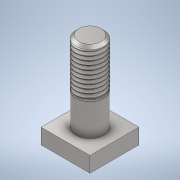
# Autodesk Inventor part: Perno de Sujeción
Saved by Autodesk Inventor 2020 (Build 240168000, 168)
## iProperties
Created: 2020-09-17
Part Number: Perno de Sujeción
Material: Steel AISI 1020 107 HR
Document SubType Name: Modeling
Designer: aaron
Density: 7.87 g/cm^3
Appearance: Stainless - Brushed
Author: aaron
Autodesk Inventor part; units mm, degrees
ref_plane "YZ Plane" through (0, 0, 0) normal (1, 0, 0) x (0, 1, 0)
ref_plane "XZ Plane" through (0, 0, 0) normal (0, 1, 0) x (-1, 0, 0)
ref_plane "XY Plane" through (0, 0, 0) normal (0, 0, 1) x (1, 0, 0)
sketch "Sketch1" plane through (0, 0, 0) normal (0, 1, 0) x (-1, 0, 0)
  line L0 (13.8906, 13.8906) -> (-13.8906, 13.8906)
  line L1 (-13.8906, 13.8906) -> (-13.8906, -13.8906)
  line L2 (-13.8906, -13.8906) -> (13.8906, -13.8906)
  line L3 (13.8906, -13.8906) -> (13.8906, 13.8906)
  line L4 (13.8906, 13.8906) -> (-13.8906, -13.8906) construction
  line L5 (-13.8906, 13.8906) -> (13.8906, -13.8906) construction
  point P0 (0, 0)
  dimension "d0" = 27.7812
  constraints: 12 end point, 2 midpoint, 2 parallel, 2 perpendicular, 1 horizontal
  measures "d0" distance of L1.end L2.end
extrude "Extrusion1" add sketch "Sketch1" against normal blind 8.7313
sketch "Sketch2" plane through (0, 0, 0) normal (0, 1, 0) x (1, 0, 0)
  circle A0 centre (0, 0) radius 7.9375
  dimension "d4" = 15.875
  constraints: 1 centre point, 1 coincident
  measures "d4" diameter of A0
extrude "Extrusion2" add sketch "Sketch2" along normal blind 45.2437
chamfer "Chamfer1" distance 1.5875 angle 45 1 edges at (-7.9375, 45.2437, 0) measured on face at (7.8347, 30.1625, 1.2733)
thread "Thread1" size "5/8-11 UNC" class "2A" standard "ANSI Unified Screw Threads" length 25.4
sketch "Sketch4" plane through (0, 43.6562, 0) normal (1, 0, 0) x (0, 0, 1)
  line L0 (7.9375, 0) -> (7.9375, 25.4)
  line L1 (7.9375, 25.4) -> (6.2254, 25.4)
  line L2 (6.2254, 25.4) -> (6.2254, 0)
  line L3 (6.2254, 0) -> (7.9375, 0)
  line L4 (0, -13.499) -> (0, 63.3686) projected
  constraints: 8 end point
revolve "Revolution1" cut sketch "Sketch4" angle 360 about axis through (0, 43.6562, 0) along (0, -1, 0)
sketch "Sketch5" plane through (0, 43.6562, 0) normal (1, 0, 0) x (0, 0, 1)
  line L0 (7.9375, 0) -> (7.9375, 25.4)
  line L1 (7.9375, 25.4) -> (6.2254, 25.4)
  line L2 (6.2254, 25.4) -> (6.2254, 0)
  line L3 (6.2254, 0) -> (7.9375, 0)
  line L4 (0, -13.499) -> (0, 63.3686) projected
  constraints: 8 end point
revolve "Revolution2" add sketch "Sketch5" angle 360 about axis through (0, 43.6562, 0) along (0, -1, 0) separate body
sketch "Sketch3" plane through (0, 43.6562, 0) normal (-1, 0, 0) x (0, -1, 0)
  line L0 (-1.3471, -6.3423) -> (-1.1546, -6.3423) construction
  line L1 (0.1923, -7.8209) -> (-0.0001, -8.1905) construction
  line L2 (-2.3092, -8.1905) -> (-2.5016, -7.8209) construction
  line L3 (-0.9622, -6.3423) -> (-1.1546, -5.9727) construction
  line L4 (-1.1546, -5.9727) -> (-1.3471, -6.3423) construction
  line L5 (-2.3092, -8.1905) -> (-2.1168, -7.8209) construction
  line L6 (-0.9622, -6.3423) -> (-0.1925, -7.8209)
  line L7 (-2.5016, -7.8209) -> (-2.1168, -7.8209) construction
  arc A0 (-2.5016, -7.8209) -> (-2.3092, -7.9377) centre (-2.3092, -7.7207) ccw construction
  line L8 (0.1923, -7.8209) -> (-0.1925, -7.8209) construction
  line L9 (-2.3092, -8.1905) -> (-2.3092, -7.8209) construction
  line L10 (-0.0001, -8.1905) -> (-0.0001, -7.8209) construction
  line L11 (-1.1546, -5.9727) -> (-1.1546, -6.2256) construction
  line L12 (-2.3092, -7.9377) -> (-0.0001, -7.9377)
  arc A1 (-2.3092, -7.9377) -> (-2.1168, -7.8209) centre (-2.3092, -7.7207) ccw
  line L13 (-0.1925, -7.8209) -> (-0.0001, -8.1905) construction
  line L14 (-2.1168, -7.8209) -> (-1.3471, -6.3423)
  line L15 (-0.0001, -0.0002) -> (-0.0001, 0.0177)
  line L16 (-0.0001, 0.0177) -> (-0.0001, -0.0002)
  line L17 (-0.0001, -0.0002) -> (0.0334, -0.0002)
  arc A2 (-0.1925, -7.8209) -> (-0.0001, -7.9377) centre (-0.0001, -7.7207) ccw
  arc A3 (-0.0001, -7.9377) -> (0.1923, -7.8209) centre (-0.0001, -7.7207) ccw construction
  arc A4 (-1.1546, -6.2256) -> (-1.3471, -6.3423) centre (-1.1546, -6.4425) ccw
  arc A5 (-0.9622, -6.3423) -> (-1.1546, -6.2256) centre (-1.1546, -6.4425) ccw
  line L18 (-1.1546, -6.2256) -> (-1.1546, -6.3423) construction
  line L19 (-1.1546, -6.3423) -> (-0.9622, -6.3423) construction
  dimension "d12" = 55
  dimension "d13" = 0.3696
  dimension "d14" = 0.3696
  dimension "Sketch3_ThreadOffset" = 0
  dimension "Sketch3_MajorRadius" = 7.9375
  dimension "d17" = 2.3091
  dimension "Sketch3_MinorRadius" = 6.2254
  constraints: 40 end point, 12 point on circle, 10 parallel, 8 tangent, 6 centre point, 6 collinear, 2 midpoint, 2 point on line, 1 horizontal, 1 perpendicular, 3 other
  measures "d12" angle of L6 L14
  measures "d13" distance of L3.end L0.end
  measures "d14" distance of L1.end L10.end
  measures "Sketch3_ThreadOffset" distance between parallel lines of L15 L10
  measures "Sketch3_MajorRadius" distance from line of L12 L15.start
  measures "d17" distance from line of L1.end L9
  measures "Sketch3_MinorRadius" distance edge to line of A5 L17
coil "Coil1" sketch "Sketch3" operation cut axis through (0, 43.6562, 0) along (0, -1, 0) pitch 2.3114 turns 12.987013 hand right bodies 2
equation "\"d12\" = d19"
equation "\"d13\" = 0.160083 * Sketch3_Pitch"
equation "\"d14\" = 0.160083 * Sketch3_Pitch"
equation "\"d17\" = Sketch3_Pitch"
equation "\"d19\" = 55deg"
equation "\"Sketch3_Pitch\" = 2.30909"
body "Solid1"
body "Solid2"
